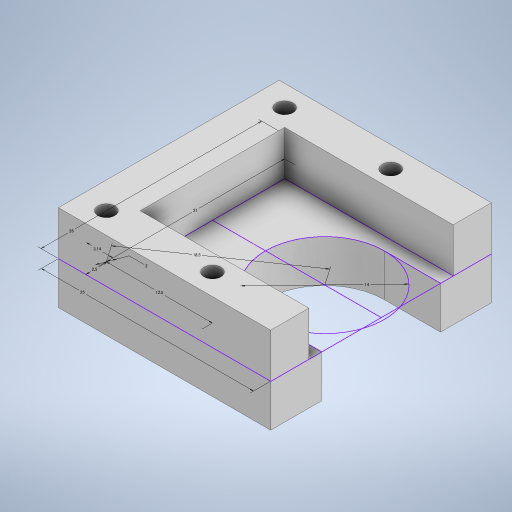
# Autodesk Inventor part: Part1
Saved by Autodesk Inventor 2024.2 (Build 282272000, 272)
## iProperties
Created: 2024-06-20
Part Number: Part1
Material: 一般
Document SubType Name: Modeling
Designer: yukin
Density: 1 g/cm^3
Appearance: 既定
Author: yukin
Autodesk Inventor part; units mm, degrees
ref_plane "YZ Plane" through (0, 0, 0) normal (1, 0, 0) x (0, 1, 0)
ref_plane "XZ Plane" through (0, 0, 0) normal (0, 1, 0) x (-1, 0, 0)
ref_plane "XY Plane" through (0, 0, 0) normal (0, 0, 1) x (1, 0, 0)
sketch "スケッチ1" plane through (0, 0, 0) normal (0, 1, 0) x (-1, 0, 0)
  line L0 (10.0552, 13) -> (-14.9448, 13)
  line L1 (-14.9448, 13) -> (-14.9448, -13)
  line L2 (-14.9448, -13) -> (10.0552, -13)
  line L3 (10.0552, -13) -> (10.0552, 13)
  line L4 (10.0552, 0) -> (-14.9448, 0)
  circle A0 centre (6.9152, 10.5) radius 1
  circle A1 centre (6.9152, 10.5) radius 2
  circle A2 centre (-5.5848, 10.5) radius 2
  circle A3 centre (-5.5848, 10.5) radius 1
  circle A4 centre (6.9152, -10.5) radius 2
  circle A5 centre (6.9152, -10.5) radius 1
  circle A6 centre (-5.5848, -10.5) radius 2
  circle A7 centre (-5.5848, -10.5) radius 1
  circle A8 centre (-8.3163, 0) radius 7
  line L5 (-8.3163, 7) -> (-14.9448, 7)
  line L6 (-8.3163, -7) -> (-14.9448, -7)
  line L7 (10.0552, 8.5) -> (-14.9448, 8.5)
  line L8 (4.9152, -13) -> (4.9152, 13)
  line L9 (10.0552, -8.5) -> (-14.9448, -8.5)
  point P0 (0, 0)
  point P1 (4.9152, 8.5)
  point P2 (4.9152, -8.5)
  point P3 (-5.5848, -8.5)
  point P4 (-5.5848, 8.5)
  dimension "d0" = 26
  dimension "d1" = 25
  dimension "d2" = 2
  dimension "d3" = 2.5
  dimension "d4" = 3.14
  dimension "d8" = 12.5
  dimension "d11" = 21
  dimension "d14" = 14
  dimension "d22" = 18.5
  constraints: 20 end point, 9 centre point, 9 point on line, 6 perpendicular, 4 coincident, 3 horizontal, 3 midpoint, 2 parallel, 2 point on circle, 2 tangent, 1 vertical, 13 other
  measures "d0" distance of L2.end L0.start
  measures "d1" distance of L0.start L0.end
  measures "d2" diameter of A0
  measures "d3" distance from line of L0 A0.centre
  measures "d4" distance from line of L3 A0.centre
  measures "d8" distance of A1.centre A2.centre
  measures "d11" distance of A1.centre A4.centre
  measures "d14" diameter of A8
  measures "d22" distance of A8.centre A1.centre
extrude "押し出し1" add sketch "スケッチ1" along normal blind 5.2 and the other way blind 5 contours L3 L7 A1 L8 L0 | A2 | L8 L7 L1 L0 | L3 L4 L8 L7 | A1 | A1 L7 L8 | L3 L9 L8 L4 | L3 L2 L8 A4 L9 | A4 | A4 L8 L9 | A6 | L8 L2 L1 L9
extrude "押し出し2" add sketch "スケッチ1" against normal blind 5 contours L3 L7 A1 L8 L0 | L8 L7 L1 L0 | L3 L4 L8 L7 | A1 L7 L8 | L3 L9 L8 L4 | L7 L8 L4 A8 L5 L1 | L3 L2 L8 A4 L9 | L8 L9 L1 L6 A8 L4 | A4 L8 L9 | L8 L2 L1 L9
